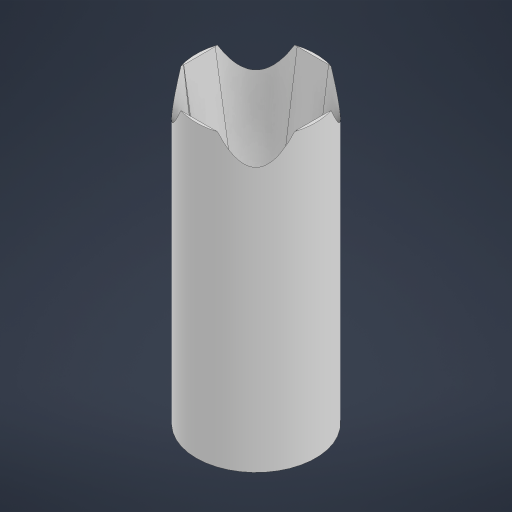
# Autodesk Inventor part: muzzle light
Saved by Autodesk Inventor 2024.3 (Build 283343000, 343)
## iProperties
Created: 2025-08-05
Part Number: muzzle light
Material: Generic
Document SubType Name: Modeling
Designer: giuseppe
Density: 1 g/cm^3
Appearance: Default
Author: giuseppe
## iProperties of the stored document muzzle light_3DPrint.ipt
Created: 2025-08-06
Part Number: muzzle light_3DPrint
Material: Generic
Document SubType Name: Modeling
Designer: giuseppe
Density: 1 g/cm^3
Appearance: Default
Author: giuseppe
Autodesk Inventor part; units mm, degrees
ref_plane "YZ Plane" through (0, 0, 0) normal (1, 0, 0) x (0, 1, 0)
ref_plane "XZ Plane" through (0, 0, 0) normal (0, 1, 0) x (-1, 0, 0)
ref_plane "XY Plane" through (0, 0, 0) normal (0, 0, 1) x (1, 0, 0)
sketch "Sketch1" plane through (0, 0, 0) normal (0, 1, 0) x (-1, 0, 0)
  circle A0 centre (0, 0) radius 9.5
  line L0 (35.7937, -26.5264) -> (-29.5588, -26.5264)
  line L1 (-29.5588, -26.5264) -> (-29.5588, 23.0689)
  line L2 (-29.5588, 23.0689) -> (35.7937, 23.0689)
  line L3 (35.7937, 23.0689) -> (35.7937, -26.5264)
  dimension "d0" = 19
  constraints: 8 end point, 2 parallel, 1 centre point, 1 coincident, 1 horizontal, 1 perpendicular
  measures "d0" diameter of A0
sketch "Sketch2" plane through (0, 0, 0) normal (0, 0, 1) x (1, 0, 0)
  line L0 (9.5, 0) -> (9.5, 53.7589) construction
  line L1 (0, 0) -> (1.5, 0) construction
  line L2 (1.5, 0) -> (9.5, 49.3559)
  line L3 (9.5, 0) -> (-9.5, 0) construction
  line L4 (1.5, 0) -> (9.5, 0)
  line L5 (9.5, 0) -> (9.5, 49.3559)
  dimension "d2" = 1.5
  dimension "d3" = 50
  constraints: 10 end point, 2 collinear, 1 horizontal, 1 point on line, 1 vertical
  measures "d2" distance of L1.start L1.end
  measures "d3" distance of L1.end L2.end
extrude "Extrusion1" add sketch "Sketch2" along normal mid plane 5
mirror "Mirror1" about plane through (0, 0, 0) normal (1, 0, 0) of "Extrusion1"
sketch "Sketch3" plane through (0, 0, 0) normal (1, 0, 0) x (0, 1, 0)
  line L0 (0, -9.5) -> (0, 9.5) projected
  line L1 (0, 9.5) -> (49.3559, 9.5)
  line L2 (0, 2.5) -> (49.3559, 2.5) projected
  line L3 (49.3559, 2.5) -> (49.3559, -2.5) projected
  line L4 (0, 2.5) -> (49.3559, 2.5) projected
  line L5 (0, -2.5) -> (0, 2.5) projected
  line L6 (49.3559, -2.5) -> (0, -2.5) projected
  line L7 (0, 2.5) -> (49.3559, 2.5) projected
  line L8 (49.3559, 9.5) -> (0, 2.5)
  line L9 (0, 9.5) -> (0, 2.5)
  point P0 (0, 0)
  constraints: 6 end point, 2 parallel, 1 collinear
extrude "Extrusion2" add sketch "Sketch3" along normal mid plane 5 contours L0 L1 L8
mirror "Mirror2" about plane through (0, 0, 0) normal (0, 0, 1) of "Extrusion2"
sketch "Sketch4" plane through (0, 0, 0) normal (0, 1, 0) x (-1, 0, 0)
  line L0 (1.5, -2.5) -> (1.5, 2.5) projected
  line L1 (1.5, -2.5) -> (9.5, -2.5) projected
  line L2 (9.5, 2.5) -> (9.5, -2.5) projected
  line L3 (9.5, 2.5) -> (1.5, 2.5) projected
  line L4 (2.5, -9.5) -> (-2.5, -9.5) projected
  line L5 (2.5, -9.5) -> (2.5, -2.5) projected
  line L6 (2.5, -2.5) -> (1.5, -2.5) projected
  line L7 (1.5, -2.5) -> (-1.5, -2.5) projected
  line L8 (-2.5, -2.5) -> (-1.5, -2.5) projected
  line L9 (-2.5, -2.5) -> (-2.5, -9.5) projected
  line L10 (-1.5, -2.5) -> (-1.5, 2.5) projected
  line L11 (-9.5, 2.5) -> (-1.5, 2.5) projected
  line L12 (-9.5, 2.5) -> (-9.5, -2.5) projected
  line L13 (-1.5, -2.5) -> (-9.5, -2.5) projected
  line L14 (2.5, 9.5) -> (-2.5, 9.5) projected
  line L15 (-2.5, 2.5) -> (-2.5, 9.5) projected
  line L16 (-1.5, 2.5) -> (-2.5, 2.5) projected
  line L17 (1.5, 2.5) -> (-1.5, 2.5) projected
  line L18 (1.5, 2.5) -> (2.5, 2.5) projected
  line L19 (2.5, 9.5) -> (2.5, 2.5) projected
  circle A0 centre (0, 0) radius 9.5 projected
  point P0 (-2.5, 9.1652)
  point P1 (-9.1652, 2.5)
  point P2 (9.1652, 2.5)
  point P3 (2.5, 9.1652)
  point P4 (-9.1652, -2.5)
  point P5 (-2.5, -9.1652)
  point P6 (2.5, -9.1652)
  point P7 (9.1652, -2.5)
extrude "Extrusion3" add sketch "Sketch4" along normal blind 46.25 contours L1 A0 L5 | L19 A0 L3 | L9 A0 L13 | L11 A0 L15
extrude "Extrusion4" cut sketch "Sketch1" along normal through all
sketch "Sketch5" plane through (0, 46.25, 0) normal (0, 1, 0) x (1, 0, 0)
  line L0 (-22.7288, -35.2268) -> (16.9474, -35.2268)
  line L1 (16.9474, -35.2268) -> (16.9474, 22.5304)
  line L2 (16.9474, 22.5304) -> (-22.7288, 22.5304)
  line L3 (-22.7288, 22.5304) -> (-22.7288, -35.2268)
  point P0 (0, 0)
  constraints: 8 end point, 2 parallel, 1 horizontal, 1 perpendicular
extrude "Extrusion5" cut sketch "Sketch5" along normal through all
sketch "Sketch6" plane through (-2.5, 6.1695, 2.5) normal (1, 0, 0) x (0, 0, -1)
  line L0 (0, -6.1695) -> (-6.5595, 40.0805) projected
  line L1 (-6.5595, 40.0805) -> (0, -6.1695) projected
  line L2 (-6.5595, 40.0805) -> (0, -6.1695) projected
  line L3 (0, 0) -> (0, -6.1695) projected
  line L4 (0, 0) -> (0, 40.0805) projected
  line L5 (-6.5595, 40.0805) -> (0, 40.0805) projected
  point P0 (2.5, -6.1695)
revolve "Revolution1" cut sketch "Sketch6" angle 90 about axis through (-2.5, 6.1695, 2.5) along (0, -1, 0)
mirror "Mirror3" about plane through (0, 0, 0) normal (1, 0, 0) of "Revolution1"
mirror "Mirror4" about plane through (0, 0, 0) normal (0, 0, 1) of "Revolution1", "Mirror3"
body "Solid1"
